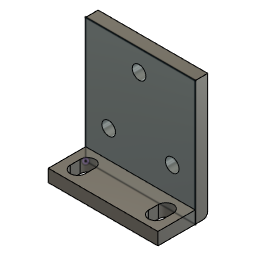
x210-24gt rack mount v6 (Autodesk Fusion 360 design; units mm, degrees)
Autodesk Fusion 360 part; units mm, degrees
sketch "スケッチ1" plane through (0, 0, 0) normal (0, 1, 0) x (1, 0, 0)
  line L0 (0, 0) -> (44, 0)
  line L1 (44, 0) -> (44, -15)
  line L2 (44, -15) -> (0, -15)
  line L3 (0, -15) -> (0, 0)
  dimension "d1" = 44
  dimension "d2" = 15
  constraint horizontal L0
  constraint vertical L1
  constraint horizontal L2
  constraint vertical L3
  constraint coincident L0.start L3.end
  measures "d1" distance of L0.start L0.end
  measures "d2" distance of L0.start L2.end
sketch "スケッチ2" plane through (0, 0, 0) normal (0, 0, 1) x (1, 0, 0)
  line L0 (0, 0) -> (44, 0)
  line L1 (44, 0) -> (44, 50)
  line L2 (44, 50) -> (0, 50)
  line L3 (0, 50) -> (0, 0)
  dimension "d3" = 44
  dimension "d4" = 50
  constraint horizontal L0
  constraint vertical L1
  constraint horizontal L2
  constraint vertical L3
  constraint coincident L0.start L3.end
  measures "d3" distance of L0.start L0.end
  measures "d4" distance of L0.start L2.end
extrude "押し出し1" add sketch "スケッチ1" along normal blind 5
extrude "押し出し2" add sketch "スケッチ2" against normal blind 5
fillet "フィレット1" radius 2 1 edges at (22, 0, -5)
sketch "スケッチ3" plane through (0, 0, 0) normal (0, 1, 0) x (1, 0, 0)
sketch "スケッチ4" plane through (0, 0, 0) normal (0, 1, 0) x (1, 0, 0)
  line L0 (6.3, -2.5) -> (6.3, -2.5)
  line L1 (9.3, -5.5) -> (9.3, -9.5)
  line L2 (6.3, -12.5) -> (6.3, -12.5)
  line L3 (3.3, -9.5) -> (3.3, -5.5)
  arc A0 (6.3, -2.5) -> (3.3, -5.5) centre (6.3, -5.5) ccw
  arc A1 (9.3, -5.5) -> (6.3, -2.5) centre (6.3, -5.5) ccw
  arc A2 (6.3, -12.5) -> (9.3, -9.5) centre (6.3, -9.5) ccw
  arc A3 (3.3, -9.5) -> (6.3, -12.5) centre (6.3, -9.5) ccw
  arc A4 (34.7, -9.5) -> (37.7, -12.5) centre (37.7, -9.5) ccw
  line L4 (37.7, -2.5) -> (37.7, -2.5)
  line L5 (34.7, -9.5) -> (34.7, -5.5)
  arc A5 (40.7, -5.5) -> (37.7, -2.5) centre (37.7, -5.5) ccw
  line L6 (40.7, -5.5) -> (40.7, -9.5)
  arc A6 (37.7, -12.5) -> (40.7, -9.5) centre (37.7, -9.5) ccw
  line L7 (37.7, -12.5) -> (37.7, -12.5)
  arc A7 (37.7, -2.5) -> (34.7, -5.5) centre (37.7, -5.5) ccw
  point P0 (3.3, -2.5)
  point P1 (9.3, -2.5)
  point P2 (3.3, -12.5)
  point P3 (34.7, -2.5)
  point P4 (40.7, -2.5)
  point P5 (34.7, -12.5)
  dimension "d11" = 6
  dimension "d12" = 10
  dimension "d13" = 3
  dimension "d14" = 6
  dimension "d15" = 10
  dimension "d16" = 3
  constraint vertical L1
  constraint vertical L3
  constraint coincident P0 L3
  constraint tangent L3 A0
  constraint coincident P1 L0
  constraint coincident P1 L1
  constraint tangent L1 A1
  constraint equal A0 A1
  constraint tangent L1 A2
  constraint equal A0 A2
  constraint coincident P2 L2
  constraint coincident P2 L3
  constraint tangent L3 A3
  constraint equal A0 A3
  constraint vertical L6
  constraint vertical L5
  constraint coincident P3 L5
  constraint tangent L5 A7
  constraint coincident P4 L4
  constraint coincident P4 L6
  constraint tangent A5 L6
  constraint equal A5 A7
  constraint tangent L6 A6
  constraint equal A6 A7
  constraint coincident P5 L7
  constraint coincident P5 L5
  constraint tangent A4 L5
  constraint equal A4 A7
  measures "d11" distance of P0 P1
  measures "d12" distance of P0 P2
  measures "d13" radius of A0
  measures "d14" distance of P3 P4
  measures "d15" distance of P3 P5
  measures "d16" radius of A7
extrude "押し出し3" cut sketch "スケッチ4" along normal blind 5
sketch "スケッチ5" plane through (0, 0, 0) normal (0, 0, 1) x (1, 0, 0)
  circle A0 centre (9.25, 16) radius 2.75
  circle A1 centre (34.75, 16) radius 2.75
  circle A2 centre (21.45, 41.581) radius 2.75
  dimension "d19" = 5.5
  dimension "d20" = 5.5
  dimension "d21" = 5.5
  measures "d19" diameter of A0
  measures "d20" diameter of A1
  measures "d21" diameter of A2
extrude "押し出し5" cut sketch "スケッチ5" against normal blind 5
extrude "押し出し4" [suppressed]
